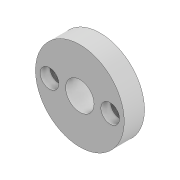
# Autodesk Inventor part: Brushless_Motor_Base
Saved by Autodesk Inventor 2020 (Build 240168000, 168)
## iProperties
Created: 2020-05-25
Part Number: Brushless_Motor_Base
Material: Generic
Document SubType Name: Modeling
Designer: Shay
Density: 1 g/cm^3
Appearance: Default
Author: Shay
Autodesk Inventor part; units mm, degrees
ref_plane "YZ Plane" through (0, 0, 0) normal (1, 0, 0) x (0, 1, 0)
ref_plane "XZ Plane" through (0, 0, 0) normal (0, 1, 0) x (-1, 0, 0)
ref_plane "XY Plane" through (0, 0, 0) normal (0, 0, 1) x (1, 0, 0)
sketch "Sketch1" plane through (0, 0, 0) normal (0, 0, 1) x (1, 0, 0)
  circle A0 centre (0, 0) radius 13.8811
  circle A1 centre (0, 0) radius 4.445
  circle A2 centre (-9.4996, 0) radius 1.7018
  circle A3 centre (9.4996, 0) radius 1.7018
  dimension "d0" = 27.7622
  dimension "d1" = 8.89
  dimension "d2" = 18.9992
  dimension "d3" = 9.4996
  dimension "d4" = 3.4036
  dimension "d5" = 3.4036
  constraints: 4 centre point, 2 coincident, 2 horizontal alignment
  measures "d0" diameter of A0
  measures "d1" diameter of A1
  measures "d2" distance of A3.centre A2.centre
  measures "d3" distance of point (0, 0) A2.centre
  measures "d4" diameter of A2
  measures "d5" diameter of A3
extrude "Extrusion1" add sketch "Sketch1" along normal blind 6.35
sketch "Sketch2" plane through (0, 0, 6.35) normal (0, 0, 1) x (1, 0, 0)
  circle A0 centre (-9.4996, 0) radius 1.7018 projected
  circle A1 centre (-9.4996, 0) radius 2.921
  circle A2 centre (9.4996, 0) radius 1.7018 projected
  circle A3 centre (9.4996, 0) radius 2.921
  point P0 (0, 0)
  dimension "d10" = 5.842
  dimension "d11" = 5.842
  constraints: 2 centre point, 2 coincident
  measures "d10" diameter of A1
  measures "d11" diameter of A3
extrude "Extrusion2" cut sketch "Sketch2" against normal blind 3.048
equation "\"d3\" = 0.5 * d2"
body "Solid1"
